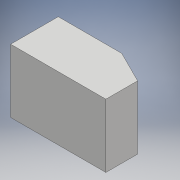
# Autodesk Inventor part: 42
Saved by Autodesk Inventor 2017 (Build 210142000, 142)
## iProperties
Part Number: 42
Material: 一般
Document SubType Name: Modeling
Designer: Brian
Density: 1 g/cm^3
Appearance: 預設
Author: Brian
Autodesk Inventor part; units mm, degrees
ref_plane "YZ Plane" through (0, 0, 0) normal (1, 0, 0) x (0, 1, 0)
ref_plane "XZ Plane" through (0, 0, 0) normal (0, 1, 0) x (-1, 0, 0)
ref_plane "XY Plane" through (0, 0, 0) normal (0, 0, 1) x (1, 0, 0)
sketch "草圖1" plane through (0, 0, 0) normal (0, 1, 0) x (-1, 0, 0)
  line L0 (0, 0) -> (-60, 0)
  line L1 (-60, 0) -> (-60, -40)
  line L2 (-60, -40) -> (0, -40)
  line L3 (0, -40) -> (0, 0)
  dimension "d0" = 40
  dimension "d1" = 60
  constraints: 8 end point, 2 parallel, 1 horizontal, 1 perpendicular
  measures "d0" distance of L2.end L0.start
  measures "d1" distance of L1.end L2.end
extrude "擠出1" add sketch "草圖1" along normal blind 20
sketch "草圖2" plane through (60, 0, -40) normal (0, 0, -1) x (-1, 0, 0)
  line L0 (60, 0) -> (60, 20) projected
  line L1 (60, 20) -> (30, 20)
  line L2 (30, 20) -> (30, 40)
  line L3 (30, 40) -> (60, 40)
  line L4 (60, 40) -> (60, 20)
  dimension "d4" = 30
  dimension "d5" = 20
  constraints: 8 end point, 2 parallel, 1 horizontal, 1 perpendicular
  measures "d4" distance of L2.end L3.end
  measures "d5" distance of L1.end L2.end
extrude "擠出2" add sketch "草圖2" against normal blind 10
sketch "草圖3" plane through (0, 0, 0) normal (0, 0, 1) x (1, 0, 0)
  line L0 (0, 20) -> (60, 20)
  line L1 (60, 20) -> (60, 30)
  line L2 (60, 30) -> (0, 30)
  line L3 (0, 30) -> (0, 20)
  line L4 (0, 20) -> (60, 20) projected
  line L5 (0, 0) -> (0, 20) projected
  dimension "d8" = 60
  dimension "d9" = 10
  constraints: 8 end point, 2 collinear, 2 parallel, 1 horizontal, 1 perpendicular
  measures "d8" distance of L1.end L2.end
  measures "d9" distance of L0.end L1.end
extrude "擠出3" add sketch "草圖3" against normal blind 10
chamfer "倒角1" distance 20 distance2 10 1 edges at (60, 30, -5) measured on face at (40, 30, -3.3333)
